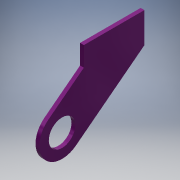
# Autodesk Inventor part: Rear roller plate
Saved by Autodesk Inventor 2017 (Build 210142000, 142)
## iProperties
Created: 2017-01-14
Part Number: Rear roller plate
Material: Generic
Document SubType Name: Modeling
Designer: Ben
Density: 1 g/cm^3
Appearance: Smooth - Purple
Author: Ben
Autodesk Inventor part; units mm, degrees
ref_plane "YZ Plane" through (0, 0, 0) normal (1, 0, 0) x (0, 1, 0)
ref_plane "XZ Plane" through (0, 0, 0) normal (0, 1, 0) x (-1, 0, 0)
ref_plane "XY Plane" through (0, 0, 0) normal (0, 0, 1) x (1, 0, 0)
sketch "Sketch1" plane through (0, 0, 0) normal (1, 0, 0) x (0, 1, 0)
  line L0 (25.4, 50.8) -> (25.4, 0)
  line L1 (25.4, 0) -> (0, 0)
  line L2 (0, 0) -> (-55.7972, 72.5494)
  line L3 (25.4, 50.8) -> (8.9951, 50.8)
  line L4 (8.9951, 50.8) -> (-25.5962, 95.7768)
  line L5 (-25.5962, 95.7768) -> (-55.7972, 72.5494)
  circle A0 centre (-29.083, 69.0626) radius 11.1125
  line L6 (-40.6967, 84.1631) -> (-29.083, 69.0626) construction
  line L7 (25.4, 25.4) -> (-19.5349, 25.4) construction
  dimension "d9" = 38.1
  dimension "d10" = 19.05
  dimension "d11" = 50.8
  dimension "d12" = 29.083
  dimension "d13" = 43.6626
  dimension "d14" = 25.4
  dimension "d16" = 22.225
  constraints: 16 end point, 3 perpendicular, 2 midpoint, 2 parallel, 1 centre point, 1 coincident, 1 horizontal, 1 point on line, 1 vertical
  measures "d9" distance of L4.end L2.end
  measures "d10" distance from line of L5 L6.end
  measures "d11" distance of L0.start L0.end
  measures "d12" horizontal distance of L6.end point (0, 0)
  measures "d13" distance from line of L6.end L7
  measures "d14" distance from line of point (0, 0) L0
  measures "d16" diameter of A0
extrude "Extrusion1" add sketch "Sketch1" along normal blind 3.175
fillet "Fillet1" radius 19.05 2 edges at (1.5875, -25.5962, 95.7768) (1.5875, -55.7972, 72.5494)
body "Solid1"
